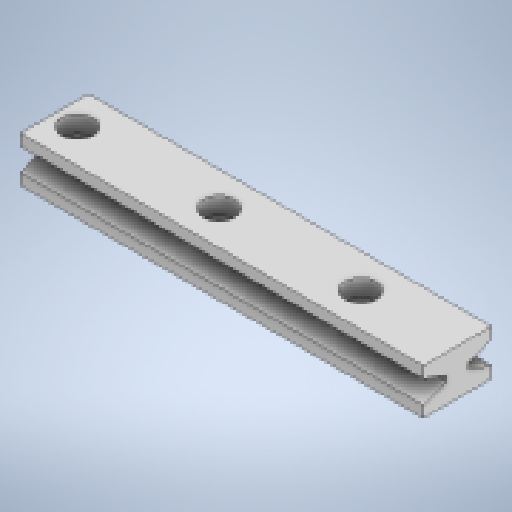
# Autodesk Inventor part: lm_guide_rail
Saved by Autodesk Inventor 2024 (Build 280153000, 153)
## iProperties
Created: 2023-09-15
Part Number: lm_guide_rail
Material: Generic
Document SubType Name: Modeling
Designer: 박동준
Density: 1 g/cm^3
Appearance: Default
Author: 박동준
Autodesk Inventor part; units mm, degrees
ref_plane "YZ Plane" through (0, 0, 0) normal (1, 0, 0) x (0, 1, 0)
ref_plane "XZ Plane" through (0, 0, 0) normal (0, 1, 0) x (-1, 0, 0)
ref_plane "XY Plane" through (0, 0, 0) normal (0, 0, 1) x (1, 0, 0)
sketch "Sketch1" plane through (0, 0, 0) normal (1, 0, 0) x (0, 1, 0)
  line L0 (-4, 6) -> (-4, -6)
  line L1 (-4, -6) -> (-2, -6)
  line L2 (2, -6) -> (4, -6)
  line L3 (4, -6) -> (4, 6)
  line L4 (4, 6) -> (2, 6)
  line L5 (2, 6) -> (0.5, 2)
  line L6 (0.5, 2) -> (-0.5, 2)
  line L7 (-0.5, 2) -> (-2, 6)
  line L8 (-2, 6) -> (-4, 6)
  line L9 (2, -6) -> (0.5, -2)
  line L10 (0.5, -2) -> (-0.5, -2)
  line L11 (-0.5, -2) -> (-2, -6)
  point P0 (0, 0)
  point P1 (-4, 0)
  point P2 (4, 0)
  point P3 (0, 2)
  point P4 (0, -2)
  dimension "d3" = 8
  dimension "d4" = 12
  dimension "d5" = 4
  dimension "d6" = 2
  dimension "d7" = 2
  dimension "d17" = 2
  dimension "d18" = 2
  dimension "d19" = 1
  dimension "d20" = 1
  dimension "d21" = 4
  constraints: 24 end point, 4 midpoint, 4 parallel, 3 perpendicular, 2 horizontal alignment, 1 collinear, 1 horizontal, 1 point on line, 1 vertical, 1 vertical alignment
  measures "d3" distance between parallel lines of L0 L3
  measures "d4" distance of L0.start L0.end
  measures "d5" distance from line of L3 point (0, 2)
  measures "d6" distance from line of L6 point (0, 0)
  measures "d7" distance of point (0, 0) point (0, -2)
  measures "d17" distance of L2.start L2.end
  measures "d18" distance of L0.end L1.end
  measures "d19" distance of L9.end L10.end
  measures "d20" distance of L5.end L6.end
  measures "d21" vertical distance of L10.end L1.end
extrude "Extrusion1" add sketch "Sketch1" along normal blind 71
sketch "Sketch2" plane through (0, 4, 6) normal (0, 1, 0) x (1, 0, 0)
  line L0 (0, 12) -> (0, 0) projected
  point P0 (0, 6)
  point P1 (4, 6)
  point P2 (29, 6)
  point P3 (0, 6)
  point P4 (0, 6)
  point P5 (54, 6)
  dimension "d22" = 4
  dimension "d23" = 25
  dimension "d31" = 25
  constraints: 2 horizontal alignment, 2 midpoint
  measures "d22" distance from line of point (4, 6) L0
  measures "d23" distance of point (29, 6) point (4, 6)
  measures "d31" distance of point (29, 6) point (54, 6)
hole "Hole1" at (4, 4, 0) at (29, 4, 0) at (54, 4, 0) direction (0, -1, 0) diameter 2.459 end through all counterbore diameter 5.5 counterbore depth 3 thread size "M3x0.5" class "6H" standard "ISO Metric profile"
body "Solid1"
